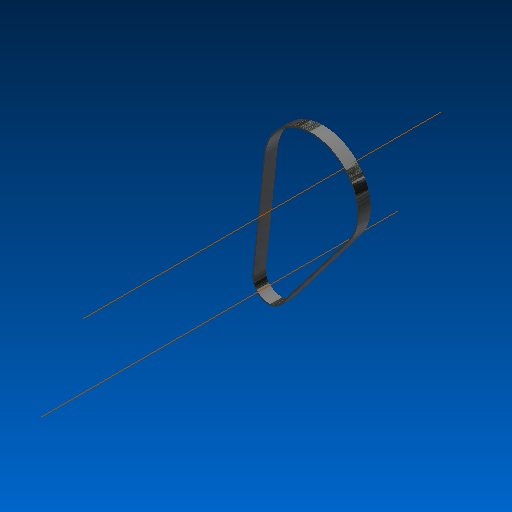
# Autodesk Inventor part: Synchronous Belt
Saved by Autodesk Inventor 2018 (Build 220112000, 112)
## iProperties
Created: 2020-07-27
Part Number: Synchronous Belt
Material: Rubber
Document SubType Name: Modeling
Designer: Bunny320
Density: 1 g/cm^3
Appearance: Rubber - Black - Version 1.1
CustomPartVersion: 1
Author: Bunny320
Autodesk Inventor part; units mm, degrees
sketch "Sketch Path" plane through (0, 0, 0) normal (0, 0, 1) x (1, 0, 0)
  arc A0 (-65.1476, -62.6009) -> (-42.3818, -71.6904) centre (-52.4861, -63.9434) ccw
  arc A1 (12.6932, 0.1427) -> (-55.604, 27.4111) centre (-17.6197, 23.3838) ccw
  line L0 (12.6932, 0.1427) -> (-42.3818, -71.6904)
  line L1 (-65.1476, -62.6009) -> (-55.604, 27.4111)
  constraints: 4 end point, 4 point on circle, 2 centre point
ref_plane "Cross Section Plane" through (-42.3818, -71.6904, 0) normal (0.6085, 0.7936, 0) x (0, 0, 1)
ref_plane "Work Plane2" through (-52.4861, -63.9434, 0) normal (-1, 0, 0) x (0, 0, 1)
ref_plane "Work Plane3" through (-17.6197, 23.3838, 0) normal (-0.1867, -0.9824, 0) x (0, 0, 1)
sketch "Cross Section" plane through (-42.3818, -71.6904, 0) normal (0.6085, 0.7936, 0) x (0, 0, 1)
  line L0 (-5, 0.5) -> (5, 0.5)
  line L1 (5, 0.5) -> (5, -0.5)
  line L2 (5, -0.5) -> (-5, -0.5)
  line L3 (-5, -0.5) -> (-5, 0.5)
  line L4 (-5, 0) -> (5, 0) construction
  point P0 (0, 0)
  point P1 (0, 0)
  dimension "d0" = 10
  dimension "d4" = 0.5
  dimension "d5" = 0.5
  constraints: 10 end point, 3 midpoint, 2 parallel, 1 coincident, 1 horizontal, 1 perpendicular, 1 other
  measures "d0" distance between parallel lines of L1 L3
  measures "d4" distance between parallel lines of L2 L4
  measures "d5" distance between parallel lines of L4 L0
sweep "Belt" add profiles "Cross Section" path "Sketch Path"
equation "\"d0\" = da_B"
equation "\"d4\" = da_a"
equation "\"d5\" = da_a2"
equation "\"da_B\" = 10"
equation "\"da_pb\" = 5"
equation "\"da_L\" = 355"
equation "\"da_a\" = 0.5"
equation "\"da_S\" = 2.65"
equation "\"da_Beta\" = 20deg"
equation "\"da_Ht\" = 1.2"
equation "\"da_H\" = 2.2"
equation "\"da_a2\" = 0.5"
body "Solid1"
